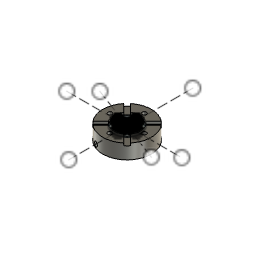
sphere_flansh_adapter v4 (Autodesk Fusion 360 design; units mm, degrees)
Autodesk Fusion 360 part; units mm, degrees
sketch "Skizze1" plane through (0, 0, 0) normal (0, 0, 1) x (1, 0, 0)
  line L0 (-49.724, 0) -> (45.1807, 0) construction
  line L1 (0, 54.1411) -> (0, -48.0834) construction
  circle A0 centre (0, 0) radius 11
  circle A1 centre (0, 0) radius 7.5 construction
  circle A2 centre (0, 0) radius 5
  circle A3 centre (0, 0) radius 1.5
  circle A4 centre (0, 7.5) radius 1.5
  circle A5 centre (7.5, 0) radius 1.5
  circle A6 centre (0, -7.5) radius 1.5
  circle A7 centre (-7.5, 0) radius 1.5
  circle A8 centre (0, 0) radius 6
  line L2 (32.1084, -12.1296) -> (-35.911, 13.566) construction
  point P0 (0, 7.5)
  point P1 (-7.5, 0)
  point P2 (0, -7.5)
  point P3 (7.5, 0)
  dimension "d1" = 22
  dimension "d2" = 15
  dimension "d3" = 10
  dimension "d4" = 3
  dimension "d9" = 3
  dimension "d10" = 3
  dimension "d11" = 3
  dimension "d12" = 3
  dimension "d22" = 12
  dimension "d117" = 20.695
  constraint horizontal L0
  constraint perpendicular L0 L1
  constraint coincident A0.centre L0
  constraint coincident A0.centre L1
  constraint coincident A0.centre A1.centre
  constraint coincident L1 P0
  constraint coincident A1 P0
  constraint coincident A1 P1
  constraint coincident L0 P1
  constraint coincident A1 P2
  constraint coincident L1 P2
  constraint coincident L0 P3
  constraint coincident A1 P3
  constraint coincident P0 A4.centre
  constraint coincident P3 A5.centre
  constraint coincident P2 A6.centre
  constraint coincident P1 A7.centre
  constraint coincident A0.centre L2
  measures "d1" diameter of A0
  measures "d2" diameter of A1
  measures "d3" diameter of A2
  measures "d4" diameter of A3
  measures "d9" diameter of A4
  measures "d10" diameter of A5
  measures "d11" diameter of A6
  measures "d12" diameter of A7
  measures "d22" diameter of A8
  measures "d117" angle of L0 L2
extrude "Extrusion1" add sketch "Skizze1" against normal blind 2 contours A0 | A8 makes body 1
extrude "Extrusion2" add sketch "Skizze1" against normal blind 12 contours A2 bodies 1
ref_plane "Arbeitsebene3" through (0, 0, 0) normal (-0.353393, -0.935475, 0) x (0.935475, -0.353393, 0)
sketch "Skizze2" plane through (0, 0, 0) normal (-0.353393, -0.935475, 0) x (-0.935475, 0.353393, 0)
  line L0 (-13.5168, 0) -> (15.568, 0) construction
  line L1 (0, -6.1401) -> (0, 17.4591) construction
  line L2 (-11.3167, 7) -> (14.0963, 7) construction
  circle A0 centre (0, 7) radius 1
  circle A1 centre (0, 7) radius 2
  point P0 (0, 7)
  dimension "d14" = 2
  dimension "d75" = 7
  dimension "d97" = 4
  constraint horizontal L0
  constraint vertical L1
  constraint coincident L1 origin
  constraint coincident L0 origin
  constraint horizontal L2
  constraint coincident L1 P0
  constraint coincident L2 P0
  constraint coincident P0 A0.centre
  measures "d14" diameter of A0
  measures "d75" distance of origin L2
  measures "d97" diameter of A1
extrude "Extrusion3" cut sketch "Skizze2" against normal blind 15 contours A0 bodies 1
ref_plane "Arbeitsebene1" through (0, 0, 10.4) normal (0, 0, 1) x (1, 0, 0)
sketch "Skizze3" plane through (0, 0, 10.4) normal (0, 0, 1) x (1, 0, 0)
  circle A0 centre (0, 0) radius 50
  circle A1 centre (0, 0) radius 7.5
  dimension "d18" = 100
  dimension "d19" = 15
  constraint coincident A0.centre A1.centre
  measures "d18" diameter of A0
  measures "d19" diameter of A1
extrude "Extrusion4" add sketch "Skizze3" along normal blind 1.6 separate body makes body 2
sketch "Skizze4" plane through (0, 0, 0) normal (0, 0, 1) x (1, 0, 0)
  circle A0 centre (0, 0) radius 5
  circle A1 centre (0, 0) radius 11
  circle A2 centre (0, 0) radius 20
  circle A3 centre (0, 0) radius 7.6
  line L0 (23.8329, 0) -> (-25.6854, 0) construction
  line L1 (0, -23) -> (0, 23) construction
  circle A4 centre (0, 0) radius 5.1
  circle A5 centre (0, 0) radius 1.5
  circle A6 centre (7.5, 0) radius 1.5 construction
  circle A7 centre (0, -7.6) radius 1.5 construction
  circle A8 centre (-7.6, 0) radius 1.5 construction
  circle A9 centre (0, 7.5) radius 1.5 construction
  line L2 (17.6858, -17.6858) -> (-21.6406, 21.6406) construction
  line L3 (17.2296, 17.2296) -> (-19.7326, -19.7326) construction
  line L4 (12.657, -15.4855) -> (3.7704, -6.5988)
  line L5 (15.4855, -12.657) -> (6.5988, -3.7704)
  line L6 (15.4855, 12.657) -> (6.5988, 3.7704)
  line L7 (12.657, 15.4855) -> (3.7704, 6.5988)
  line L8 (-12.657, 15.4855) -> (-3.7704, 6.5988)
  line L9 (-15.4855, 12.657) -> (-6.5988, 3.7704)
  line L10 (-12.657, -15.4855) -> (-3.7704, -6.5988)
  line L11 (-15.4855, -12.657) -> (-6.5988, -3.7704)
  circle A10 centre (0, 0) radius 11
  circle A11 centre (0, 0) radius 8 construction
  circle A12 centre (8, 0) radius 1.25
  circle A13 centre (0, 8) radius 1.25
  circle A14 centre (-8, 0) radius 1.25
  circle A15 centre (0, -8) radius 1.25
  line L12 (5.9, -1.2124) -> (8, -2.4249)
  line L13 (8, -2.4249) -> (10.1, -1.2124)
  line L14 (10.1, -1.2124) -> (10.1, 1.2124)
  line L15 (10.1, 1.2124) -> (8, 2.4249)
  line L16 (8, 2.4249) -> (5.9, 1.2124)
  line L17 (5.9, 1.2124) -> (5.9, -1.2124)
  line L18 (21.0556, -6.9134) -> (-8.44, 22.5822) construction
  circle A16 centre (0, 0) radius 14.1421 construction
  circle A17 centre (14.1421, 0) radius 1.75
  line L19 (16.9921, 1.6454) -> (14.1421, 3.2909) construction
  line L20 (14.1421, 3.2909) -> (11.2921, 1.6454) construction
  line L21 (11.2921, 1.6454) -> (11.2921, -1.6454) construction
  line L22 (11.2921, -1.6454) -> (14.1421, -3.2909) construction
  line L23 (14.1421, -3.2909) -> (16.9921, -1.6454) construction
  line L24 (16.9921, -1.6454) -> (16.9921, 1.6454) construction
  circle A18 centre (0, -14.1421) radius 1.75
  circle A19 centre (-14.1421, 0) radius 1.75
  circle A20 centre (0, 14.1421) radius 1.75
  circle A21 centre (0, 8) radius 2
  circle A22 centre (-8, 0) radius 2
  circle A23 centre (0, -8) radius 2
  circle A24 centre (8, 0) radius 2
  point P0 (0, -7.6)
  point P1 (-7.6, 0)
  point P2 (0, 7.6)
  point P3 (7.6, 0)
  point P4 (0, 8)
  point P5 (-8, 0)
  point P6 (0, -8)
  point P7 (8, 0)
  point P8 (8, 0)
  point P9 (0, 14.1421)
  point P10 (14.1421, 0)
  point P11 (0, -14.1421)
  point P12 (-14.1421, 0)
  point P13 (14.1421, 0)
  dimension "d31" = 40
  dimension "d32" = 15.2
  dimension "d37" = 10.2
  dimension "d42" = 3
  dimension "d47" = 3
  dimension "d48" = 3
  dimension "d49" = 3
  dimension "d50" = 3
  dimension "d63" = 45
  dimension "d64" = 45
  dimension "d65" = 2
  dimension "d66" = 2
  dimension "d67" = 2
  dimension "d68" = 2
  dimension "d69" = 2
  dimension "d70" = 2
  dimension "d71" = 2
  dimension "d72" = 2
  dimension "d76" = 22
  dimension "d77" = 16
  dimension "d78" = 2.5
  dimension "d79" = 2.5
  dimension "d80" = 2.5
  dimension "d81" = 2.5
  dimension "d82" = 4.2
  dimension "d90" = 10
  dimension "d91" = 28.2843
  dimension "d92" = 3.5
  dimension "d93" = 5.7
  dimension "d94" = 3.5
  dimension "d95" = 3.5
  dimension "d96" = 3.5
  dimension "d100" = 4
  dimension "d101" = 4
  dimension "d102" = 4
  dimension "d103" = 4
  constraint coincident A0.centre A1.centre
  constraint coincident A0.centre L1
  constraint coincident A0.centre L0
  constraint coincident A3 P0
  constraint coincident L1 P0
  constraint coincident A3 P1
  constraint coincident L0 P1
  constraint coincident A3 P2
  constraint coincident L1 P2
  constraint coincident L0 P3
  constraint coincident A3 P3
  constraint coincident P0 A7.centre
  constraint coincident P1 A8.centre
  constraint coincident A0.centre L3
  constraint coincident A0.centre L2
  constraint perpendicular L0 L1
  constraint horizontal L0
  constraint parallel L3 L11
  constraint parallel L3 L10
  constraint parallel L2 L4
  constraint parallel L2 L5
  constraint parallel L3 L6
  constraint parallel L3 L7
  constraint parallel L2 L8
  constraint parallel L2 L9
  constraint coincident A3 L9.end
  constraint coincident A3 L8.end
  constraint coincident A3 L7.end
  constraint coincident A3 L6.end
  constraint coincident A3 L5.end
  constraint coincident A3 L4.end
  constraint coincident A3 L10.end
  constraint coincident A3 L11.end
  constraint coincident A2 L9.start
  constraint coincident A2 L8.start
  constraint coincident A2 L7.start
  constraint coincident A2 L6.start
  constraint coincident A2 L5.start
  constraint coincident A2 L4.start
  constraint coincident A2 L10.start
  constraint coincident A2 L11.start
  constraint coincident A11 P4
  constraint coincident L1 P4
  constraint coincident A11 P5
  constraint coincident L0 P5
  constraint coincident L1 P6
  constraint coincident A11 P6
  constraint coincident L0 P8
  constraint coincident A11 P8
  constraint coincident P8 P7
  constraint coincident P4 A13.centre
  constraint coincident P5 A14.centre
  constraint coincident P6 A15.centre
  constraint perpendicular L3 L18
  constraint coincident L1 P9
  constraint coincident L18 P9
  constraint coincident P9 A16
  constraint coincident L0 P13
  constraint coincident L18 P13
  constraint coincident A16 P11
  constraint coincident L1 P11
  constraint coincident L0 P12
  constraint coincident A16 P12
  constraint coincident P13 P10
  constraint coincident P11 A18.centre
  constraint coincident P12 A19.centre
  constraint coincident P9 A20.centre
  measures "d31" diameter of A2
  measures "d32" diameter of A3
  measures "d37" diameter of A4
  measures "d42" diameter of A5
  measures "d47" diameter of A9
  measures "d48" diameter of A6
  measures "d49" diameter of A7
  measures "d50" diameter of A8
  measures "d63" angle of L1 L2
  measures "d64" angle of L1 L3
  measures "d65" distance of L2 L9
  measures "d66" distance of L2 L8
  measures "d67" distance of L3 L11
  measures "d68" distance of L3 L10
  measures "d69" distance of L2 L4
  measures "d70" distance of L2 L5
  measures "d71" distance of L3 L6
  measures "d72" distance of L3 L7
  measures "d76" diameter of A10
  measures "d77" diameter of A11
  measures "d78" diameter of A12
  measures "d79" diameter of A13
  measures "d80" diameter of A14
  measures "d81" diameter of A15
  measures "d82" distance of L14 L17
  measures "d90" distance of A0.centre L18
  measures "d91" diameter of A16
  measures "d92" diameter of A17
  measures "d93" distance of L21 L24
  measures "d94" diameter of A18
  measures "d95" diameter of A19
  measures "d96" diameter of A20
  measures "d100" diameter of A21
  measures "d101" diameter of A22
  measures "d102" diameter of A23
  measures "d103" diameter of A24
extrude "Extrusion11" add sketch "Skizze4" along normal blind 2 separate body contours A1 A2 L5 L6 A10 | A1 A2 L7 L8 A10 | A1 A2 L4 L10 A10 | A1 A2 L9 L11 A10 makes body 3 at (-4.9039, -14.0965, 0) makes body 4 at (14.1401, 4.9023, 2) makes body 5 at (-14.1401, 4.9023, 0) makes body 6 at (4.9039, 14.0965, 0)
extrude "Extrusion12" add sketch "Skizze4" against normal blind 10 contours A1 A3 L5 L6 A10 L12 L13 L14 L15 L16 | A1 A2 L5 L6 A10 | A1 A3 L6 L7 A10 | A1 A2 L6 L7 A10 | A1 A2 L4 L5 A10 | A1 A3 L4 L5 A10 | A1 A3 L7 L8 A10 A21 | A1 A2 L7 L8 A10 | A3 L12 L16 L17 A21 A22 A23 | A1 A2 L4 L10 A10 | A1 A3 L4 L10 A10 A23 | A1 A3 L8 L9 A10 | A1 A2 L8 L9 A10 | A3 L12 L13 L14 L15 L16 A24 | A3 L12 L16 L17 A24 | A1 A2 L10 L11 A10 | A1 A3 L10 L11 A10 | A1 A3 L9 L11 A10 A22 | A1 A2 L9 L11 A10 bodies 3 4 5 6
extrude "Extrusion15" add sketch "Skizze4" against normal blind 4 contours A3 A13 A21 | A3 A13 A21 | A3 A12 A24 | A3 A12 A24 | A3 A15 A23 | A3 A15 A23 | A3 A14 A22 | A3 A14 A22 bodies 3
extrude "Extrusion13" cut sketch "Skizze4" against normal blind 2 contours A1 A3 L5 L6 A10 L12 L13 L14 L15 L16 | A1 A3 L6 L7 A10 | A1 A3 L4 L5 A10 | A1 A3 L7 L8 A10 A21 | A3 L12 L16 L17 A21 A22 A23 | A1 A3 L4 L10 A10 A23 | A1 A3 L8 L9 A10 | A3 L12 L13 L14 L15 L16 A24 | A3 L12 L16 L17 A24 | A1 A3 L10 L11 A10 | A1 A3 L9 L11 A10 A22 | A3 A13 A21 | A3 A13 A21 | A3 A12 A24 | A3 A12 A24 | A3 A15 A23 | A3 A15 A23 | A3 A14 A22 | A3 A14 A22 bodies 3
extrude "Extrusion14" cut sketch "Skizze2" along normal mid plane 60 contours A0 | A1 bodies 3
ref_plane "Arbeitsebene2" through (0, 0, -1) normal (0, 0, 1) x (1, 0, 0)
sketch "Skizze5" plane through (0, 0, -1) normal (0, 0, 1) x (1, 0, 0)
  line L0 (-26, 0) -> (29, 0) construction
  line L1 (0, 26.6665) -> (0, -26.3793) construction
  circle A0 centre (0, 0) radius 14.142 construction
  line L2 (-1.6454, 16.992) -> (-3.2909, 14.142)
  line L3 (-3.2909, 14.142) -> (-1.6454, 11.292)
  line L4 (-1.6454, 11.292) -> (1.6454, 11.292)
  line L5 (1.6454, 11.292) -> (3.2909, 14.142)
  line L6 (3.2909, 14.142) -> (1.6454, 16.992)
  line L7 (1.6454, 16.992) -> (-1.6454, 16.992)
  line L8 (16.992, 1.6454) -> (14.142, 3.2909)
  line L9 (14.142, 3.2909) -> (11.292, 1.6454)
  line L10 (11.292, 1.6454) -> (11.292, -1.6454)
  line L11 (11.292, -1.6454) -> (14.142, -3.2909)
  line L12 (14.142, -3.2909) -> (16.992, -1.6454)
  line L13 (16.992, -1.6454) -> (16.992, 1.6454)
  line L14 (1.6454, -16.992) -> (3.2909, -14.142)
  line L15 (3.2909, -14.142) -> (1.6454, -11.292)
  line L16 (1.6454, -11.292) -> (-1.6454, -11.292)
  line L17 (-1.6454, -11.292) -> (-3.2909, -14.142)
  line L18 (-3.2909, -14.142) -> (-1.6454, -16.992)
  line L19 (-1.6454, -16.992) -> (1.6454, -16.992)
  line L20 (-16.992, -1.6454) -> (-14.142, -3.2909)
  line L21 (-14.142, -3.2909) -> (-11.292, -1.6454)
  line L22 (-11.292, -1.6454) -> (-11.292, 1.6454)
  line L23 (-11.292, 1.6454) -> (-14.142, 3.2909)
  line L24 (-14.142, 3.2909) -> (-16.992, 1.6454)
  line L25 (-16.992, 1.6454) -> (-16.992, -1.6454)
  point P0 (0, 14.142)
  point P1 (-14.142, 0)
  point P2 (0, -14.142)
  point P3 (14.142, 0)
  point P4 (0, 14.142)
  point P5 (14.142, 0)
  point P6 (0, -14.142)
  point P7 (-14.142, 0)
  dimension "d107" = 28.284
  dimension "d108" = 5.7
  dimension "d109" = 5.7
  dimension "d110" = 5.7
  dimension "d111" = 5.7
  constraint horizontal L0
  constraint vertical L1
  constraint coincident A0.centre L1
  constraint coincident A0.centre L0
  constraint coincident A0.centre origin
  constraint coincident A0 P4
  constraint coincident L1 P4
  constraint coincident A0 P1
  constraint coincident L0 P1
  constraint coincident L1 P6
  constraint coincident A0 P6
  constraint coincident A0 P5
  constraint coincident L0 P5
  constraint coincident P4 P0
  constraint coincident P5 P3
  constraint coincident P6 P2
  constraint coincident P1 P7
  measures "d107" diameter of A0
  measures "d108" distance of L4 L7
  measures "d109" distance of L10 L13
  measures "d110" distance of L16 L19
  measures "d111" distance of L22 L25
extrude "Extrusion16" cut sketch "Skizze5" against normal blind 2.6 bodies 3
hidden bodies 1 2
named bodies: "Flanschkupplung", "pcb", "Adapter"
